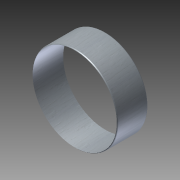
# Autodesk Inventor part: Duct_Outer
Saved by Autodesk Inventor 2011 SP1 (Build 150282100, 282)
## iProperties
Created: 2011-06-11
Part Number: Duct_Outer
Document SubType Name: Modeling
Designer: Andrew G. Meyer
Mass: 78.5492 g
Surface Area: 1018.34 cm^2
Volume: 78.5492 cm^3
Density: 1 g/cm^3
Author: Andrew G. Meyer
Autodesk Inventor part; units mm, degrees
ref_plane "YZ Plane" through (0, 0, 0) normal (1, 0, 0) x (0, 1, 0)
ref_plane "XZ Plane" through (0, 0, 0) normal (0, 1, 0) x (-1, 0, 0)
ref_plane "XY Plane" through (0, 0, 0) normal (0, 0, 1) x (1, 0, 0)
sketch "Sketch1" plane through (0, 0, 0) normal (0, 0, 1) x (1, 0, 0)
  circle A0 centre (0, 0) radius 104.775
  circle A1 centre (0, 0) radius 106.3625
  dimension "d0" = 1.5875
  dimension "d1" = 209.55
  constraints: 2 centre point, 2 coincident
  measures "d0" radial gap between concentric circles of A1 A0
  measures "d1" diameter of A0
extrude "Extrusion1" add sketch "Sketch1" along normal blind 76.2
fillet "Fillet1" radius 3.175 2 edges at (-106.3625, 0, 76.2) (-106.3625, 0, 0)
body "Solid1"
